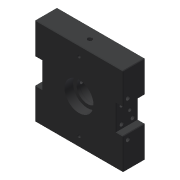
# Autodesk Inventor part: middleplate
Saved by Autodesk Inventor 2022 Beta2 (Build 260130000, 130) ContinuousBuild 0
## iProperties
Shininess: 64.0
Length Units: 11269
Angle Units: 11279
Time Units: 11290
Mass Units: 11283
Length Display Precision: 3
Angle Display Precision: 2
Compacted: True
Part Number: middleplate
Document SubType Name: Modeling
Created: 2003-04-03
Designer: Sudhir John
Density: 1 g/cm^3
Material: Generic
Appearance: Generic
Density: 0.0
Volumn: 0.0
Area: 0.0
PropertySet Name: Model Information
Control State: 0
Master: False
Checked Out: False
Author: Sudhir John
Autodesk Inventor part; units mm, degrees
sketch "Sketch1" plane through (0, 0, 0) normal (0, 0, 1) x (1, 0, 0)
  line L0 (-13.4367, -170.0605) -> (189.7633, -170.0605)
  line L1 (189.7633, -170.0605) -> (189.7633, 33.1395)
  line L2 (189.7633, 33.1395) -> (-13.4367, 33.1395)
  line L3 (-13.4367, 33.1395) -> (-13.4367, -170.0605)
  dimension "d0" = 203.2
  dimension "d1" = 203.2
  constraints: 8 end point, 2 parallel, 1 horizontal, 1 perpendicular
  measures "d0" distance of L1.end L2.end
  measures "d1" distance of L2.end L0.start
extrude "Extrusion1" add sketch "Sketch1" along normal blind 50.8
ref_plane "Work Plane1" through (88.1633, -170.0605, 0) normal (1, 0, 0) x (0, 0, -1)
ref_plane "Work Plane2" through (-13.4367, -68.4605, 0) normal (0, 1, 0) x (1, 0, 0)
sketch "Sketch2" plane through (0, 0, 50.8) normal (0, 0, 1) x (1, 0, 0)
  line L0 (-13.4367, -170.0605) -> (-13.4367, 33.1395) projected
  line L1 (-13.4367, -39.8855) -> (2.5653, -39.8855)
  line L2 (2.5653, -39.8855) -> (2.5653, -97.0355)
  line L3 (2.5653, -97.0355) -> (-13.4367, -97.0355)
  line L4 (-13.4367, -97.0355) -> (-13.4367, -39.8855)
  line L5 (-33.7567, -68.4605) -> (250.7233, -68.4605) projected
  dimension "d4" = 16.002
  dimension "d5" = 57.15
  dimension "d6" = 28.575
  constraints: 8 end point, 2 parallel, 1 horizontal, 1 perpendicular, 1 point on line
  measures "d4" distance of L1.start L1.end
  measures "d5" distance of L1.end L2.end
  measures "d6" distance between parallel lines of L1 L5
extrude "Extrusion2" cut sketch "Sketch2" against normal through all
mirror "Mirror1" about plane through (88.1633, -170.0605, 0) normal (1, 0, 0) of "Extrusion2"
sketch "Sketch3" plane through (-13.4367, -68.4605, 0) normal (0, 1, 0) x (1, 0, 0)
  line L0 (101.6, 5.08) -> (101.6, -66.04) projected
  line L1 (101.6, -50.8) -> (134.9502, -50.8)
  line L2 (134.9502, -50.8) -> (134.9502, -31.115)
  line L3 (134.9502, -31.115) -> (126.7758, -31.115)
  line L4 (126.7758, -31.115) -> (126.7758, -24.8158)
  line L5 (126.7758, -24.8158) -> (127.135, -23.4478)
  line L6 (127.135, -23.4478) -> (127.135, -6.3536)
  line L7 (127.135, -6.3536) -> (127.2293, -5.9944)
  line L8 (127.2293, -5.9944) -> (131.7752, -5.9944)
  line L9 (131.7752, -5.9944) -> (131.7752, 0)
  line L10 (131.7752, 0) -> (101.6, 0)
  line L11 (203.2, 0) -> (0, 0) projected
  line L12 (0, -50.8) -> (203.2, -50.8) projected
  point P0 (131.7752, -2.9972)
  dimension "d9" = 30.1752
  dimension "d10" = 5.9944
  dimension "d11" = 17.0942
  dimension "d12" = 6.2992
  dimension "d13" = 19.685
  dimension "d14" = 33.3502
  constraints: 20 end point, 5 parallel, 3 perpendicular, 2 collinear, 2 point on line, 1 midpoint, 1 vertical
  measures "d9" distance between parallel lines of L0 L9
  measures "d10" distance of L8.end L9.end
  measures "d11" distance of L5.end L6.end
  measures "d12" distance of L3.end L4.end
  measures "d13" distance of L1.end L2.end
  measures "d14" distance of L1.start L1.end
revolve "Revolution1" cut sketch "Sketch3" angle 360 about axis through (88.1633, -68.4605, 0) along (0, 0, 1)
sketch "Sketch6" plane through (-13.4367, -170.0605, 0) normal (0, -1, 0) x (1, 0, 0)
  line L0 (76.2, 50.8) -> (0, 50.8) projected
  line L1 (101.6, 66.04) -> (101.6, -5.08) projected
  point P0 (60.325, 19.05)
  point P1 (142.875, 19.05)
  dimension "d31" = 41.275
  dimension "d32" = 31.75
  constraints: 1 symmetric about line
  measures "d31" distance from line of L1 point (60.325, 19.05)
  measures "d32" distance from line of L0 point (60.325, 19.05)
hole "Hole2" at (46.8883, -170.0605, 19.05) at (129.4383, -170.0605, 19.05) direction (0, 1, 0) diameter 8.7122 depth 85.5726 tip angle 118 counterbore diameter 19.05 counterbore depth 5.08
sketch "Sketch7" plane through (189.7633, -170.0605, 50.8) normal (1, 0, 0) x (0, 0, -1)
  line L0 (0, 73.025) -> (0, 0) projected
  line L1 (-15.24, 101.6) -> (55.88, 101.6) projected
  point P0 (11.176, 60.325)
  point P1 (11.176, 142.875)
  dimension "d40" = 41.275
  dimension "d41" = 11.176
  constraints: 1 symmetric about line
  measures "d40" distance from line of L1 point (11.176, 60.325)
  measures "d41" distance from line of L0 point (11.176, 60.325)
hole "Hole3" at (189.7633, -109.7355, 39.624) at (189.7633, -27.1855, 39.624) direction (-1, 0, 0) diameter 9.144 depth 32.4612 tip angle 118 thread size "7/16-14 UNC" class "1B" standard "ANSI Unified Screw Threads"
mirror "Mirror3" about plane through (88.1633, -170.0605, 0) normal (1, 0, 0) of "Hole3"
ref_plane "Work Plane3" through (0, 0, 25.4) normal (0, 0, 1) x (1, 0, 0)
sketch "Sketch8" plane through (173.7613, -97.0355, 0) normal (1, 0, 0) x (0, 0, -1)
  line L0 (-25.4, -93.345) -> (-25.4, 191.135) projected
  line L1 (-66.04, 28.575) -> (5.08, 28.575) projected
  point P0 (-38.1, 47.625)
  point P1 (-12.7, 47.625)
  point P2 (-38.1, 9.525)
  point P3 (-12.7, 9.525)
  dimension "d49" = 12.7
  dimension "d50" = 19.05
  constraints: 3 symmetric about line
  measures "d49" distance from line of L0 point (-38.1, 47.625)
  measures "d50" distance from line of L1 point (-38.1, 47.625)
hole "Hole4" at (173.7613, -49.4105, 38.1) at (173.7613, -49.4105, 12.7) at (173.7613, -87.5105, 38.1) at (173.7613, -87.5105, 12.7) direction (-1, 0, 0) diameter 9.144 depth 18.8468 tip angle 118 thread size "7/16-14 UNC" class "1B" standard "ANSI Unified Screw Threads"
mirror "Mirror4" about plane through (88.1633, -170.0605, 0) normal (1, 0, 0) of "Hole4"
sketch "Sketch9" plane through (0, 0, 0) normal (0, 0, -1) x (-1, 0, 0)
  line L0 (-189.7633, 33.1395) -> (13.4367, 33.1395) projected
  line L1 (-250.7233, -68.4605) -> (33.7567, -68.4605) projected
  point P0 (-88.1633, 11.0415)
  point P1 (-88.1633, -147.9625)
  dimension "d58" = 22.098
  constraints: 1 symmetric about line
  measures "d58" distance from line of L0 point (-88.163, 11.042)
hole "Hole5" at (88.1633, 11.0415, 0) at (88.1633, -147.9625, 0) direction (0, 0, 1) diameter 7.1374 end through all counterbore diameter 10.3124 counterbore depth 8.128
sketch "Sketch10" plane through (173.7613, -97.0355, 0) normal (1, 0, 0) x (0, 0, -1)
  line L0 (0, 57.15) -> (0, 0) projected
  point P0 (-19.0754, 28.575)
  dimension "d66" = 19.0754
  measures "d66" distance from line of L0 point (-19.075, 28.575)
hole "Hole6" at (173.7613, -68.4605, 19.0754) direction (-1, 0, 0) diameter 7.7978 depth 128.7018 tip angle 118 thread size "3/8-16 UNC" class "1B" standard "ANSI Unified Screw Threads"
sketch "Sketch11" plane through (-13.4367, 33.1395, 0) normal (0, 1, 0) x (1, 0, 0)
  line L0 (203.2, 0) -> (0, 0) projected
  line L1 (101.6, 5.08) -> (101.6, -66.04) projected
  point P0 (101.6, -25.3924)
  dimension "d74" = 25.3924
  constraints: 1 point on line
  measures "d74" distance from line of L0 point (101.6, -25.392)
hole "Hole7" at (88.1633, 33.1395, 25.3924) direction (0, -1, 0) diameter 10.414 depth 32.258 tip angle 118 thread size "1/2-12 UNS" class "2B" standard "ANSI Unified Screw Threads"
mirror "Mirror5" about plane through (-13.4367, -68.4605, 0) normal (0, 1, 0) of "Hole7"
chamfer "Chamfer1" distance 1.27 angle 45 32 edges at (88.1633, 33.1395, 50.8) (189.7633, 33.1395, 25.4) (189.7633, -3.373, 50.8) (189.7633, -3.373, 0) (189.7633, -39.8855, 25.4) (181.7623, -39.8855, 50.8) (173.7613, -68.4605, 50.8) (181.7623, -97.0355, 50.8) (189.7633, -97.0355, 25.4) (189.7633, -133.548, 50.8) (189.7633, -133.548, 0) (189.7633, -170.0605, 25.4) (88.1633, -170.0605, 50.8) (-13.4367, -170.0605, 25.4) (-13.4367, -133.548, 50.8) (-5.4357, -97.0355, 50.8) (2.5653, -68.4605, 50.8) (-5.4357, -39.8855, 50.8) (-13.4367, -3.373, 50.8) (-13.4367, -97.0355, 25.4) (-13.4367, -39.8855, 25.4) (-13.4367, 33.1395, 25.4) (88.1633, 33.1395, 0) (181.7623, -39.8855, 0) (173.7613, -68.4605, 0) (181.7623, -97.0355, 0) (-5.4357, -97.0355, 0) (2.5653, -68.4605, 0) (-5.4357, -39.8855, 0) (-13.4367, -3.373, 0) (88.1633, -170.0605, 0) (-13.4367, -133.548, 0)
body "Solid1"
